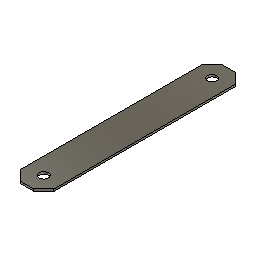
LumenPnPStagingPlateSpacer (Autodesk Fusion 360 design; units mm, degrees)
Autodesk Fusion 360 part; units mm, degrees
sketch "Sketch1" plane through (0, 0, 0) normal (0, 0, 1) x (1, 0, 0)
  line L0 (-10, 60) -> (10, 60)
  line L1 (10, 60) -> (10, -60)
  line L2 (10, -60) -> (-10, -60)
  line L3 (-10, -60) -> (-10, 60)
  line L4 (-10, 60) -> (10, -60) construction
  line L5 (10, 60) -> (-10, -60) construction
  circle A0 centre (0, -50) radius 2.7
  line L6 (0, -50) -> (-10, -50) construction
  line L7 (0, -50) -> (0, -60) construction
  line L8 (90, 0) -> (-64.2965, 0) construction
  circle A1 centre (0, 50) radius 2.7
  dimension "d1" = 120
  dimension "d2" = 20
  dimension "d3" = 5.4
  constraint horizontal L0
  constraint perpendicular L0 L1
  constraint parallel L0 L2
  constraint parallel L1 L3
  constraint coincident L4 origin
  constraint coincident L5 origin
  constraint coincident A0.centre L6.start
  constraint coincident L3 L6.end
  constraint perpendicular L3 L6
  constraint midpoint L2 L7.end
  constraint vertical L7
  constraint equal L6 L7
  constraint horizontal L8
  constraint symmetric A0 L8 A1
  measures "d1" distance of L0.end L1.end
  measures "d2" distance of L1.end L2.end
  measures "d3" diameter of A0
extrude "Extrude1" add sketch "Sketch1" along normal blind 1.2
chamfer "Chamfer1" distance 6 angle 45 2 edges at (10, -60, 0.6) (-10, -60, 0.6)
chamfer "Chamfer1" distance 6 angle 45 2 edges at (10, 60, 0.6) (-10, 60, 0.6)
